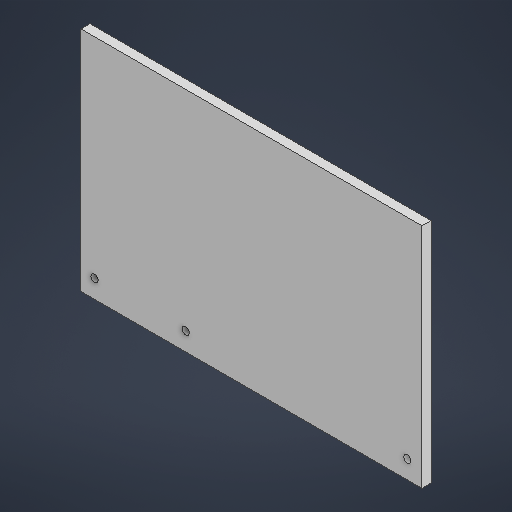
# Autodesk Inventor part: крепление сосала
Saved by Autodesk Inventor 2026.2 (Build 302298000, 298)
## iProperties
Created: 2026-01-20
Part Number: крепление сосала
Material: Типовые
Document SubType Name: Modeling
Designer: Phantom
Density: 1 g/cm^3
Appearance: По умолчанию
Author: Phantom
Autodesk Inventor part; units mm, degrees
ref_plane "YZ Plane" through (0, 0, 0) normal (1, 0, 0) x (0, 1, 0)
ref_plane "XZ Plane" through (0, 0, 0) normal (0, 1, 0) x (-1, 0, 0)
ref_plane "XY Plane" through (0, 0, 0) normal (0, 0, 1) x (1, 0, 0)
sketch "Эскиз1" plane through (0, 0, 0) normal (0, 0, 1) x (1, 0, 0)
  line L0 (0, 0) -> (150, 0)
  line L1 (150, 0) -> (150, 100)
  line L2 (150, 100) -> (0, 100)
  line L3 (0, 100) -> (0, 0)
  circle A0 centre (46.1, 8) radius 1.625
  circle A1 centre (143.5763, 8) radius 1.625
  circle A2 centre (6, 8) radius 1.625
  line L4 (6, 8) -> (143.5763, 8)
  dimension "d0" = 150
  dimension "d1" = 100
  dimension "d2" = 97.4763
  dimension "d3" = 40.1
  dimension "d4" = 8
  dimension "d5" = 6
  constraints: 10 end point, 3 centre point, 2 horizontal, 2 parallel, 1 perpendicular
  measures "d0" distance of L2.end L1.end
  measures "d1" distance of L1.end L0.end
  measures "d2" distance of A0.centre L4.end
  measures "d3" distance of L4.start A0.centre
  measures "d4" distance between parallel lines of L0 L4
  measures "d5" distance from line of L3 L4.start
extrude "Выдавливание1" add sketch "Эскиз1" along normal blind 4
